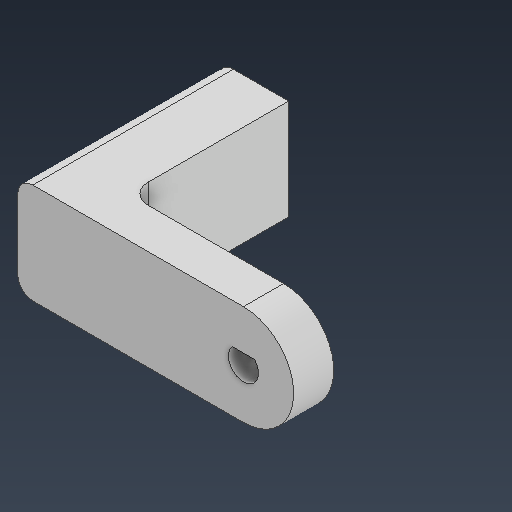
# Autodesk Inventor part: AcoplePPR
Saved by Autodesk Inventor 2027 (Build 310192000, 192)
## iProperties
Created: 2026-08-17
Part Number: AcoplePPR
Material: Generic
Document SubType Name: Modeling
Designer: 06aar
Density: 1 g/cm^3
Appearance: Default
Author: 06aar
Autodesk Inventor part; units mm, degrees
ref_plane "YZ Plane" through (0, 0, 0) normal (1, 0, 0) x (0, 1, 0)
ref_plane "XZ Plane" through (0, 0, 0) normal (0, 1, 0) x (-1, 0, 0)
ref_plane "XY Plane" through (0, 0, 0) normal (0, 0, 1) x (1, 0, 0)
sketch "Sketch1" plane through (0, 0, 0) normal (0, 0, 1) x (1, 0, 0)
  circle A0 centre (0, 0) radius 1.5
  circle A1 centre (0, 0) radius 5
  line L0 (0, 5) -> (-17.5, 5)
  circle A2 centre (-17.5, 0) radius 5
  line L1 (-17.5, -5) -> (0, -5)
  line L2 (-17.5, 0) -> (0, 0)
  line L3 (-17.5, 5) -> (-22.5, 5)
  line L4 (-22.5, 5) -> (-22.5, -5)
  line L5 (-22.5, -5) -> (-17.5, -5)
  line L6 (-1.118, 1) -> (1.118, 1)
  line L7 (0, 1) -> (0, -1.5)
  point P0 (-22.5, 0)
  dimension "d0" = 3
  dimension "d1" = 3.5
  dimension "d3" = 17.5
  dimension "d12" = 2.5
  constraints: 16 end point, 7 point on circle, 6 tangent, 4 horizontal, 3 centre point, 2 coincident, 2 perpendicular, 1 midpoint, 1 parallel, 1 vertical
  measures "d0" diameter of A0
  measures "d1" radial gap between concentric circles of A0 A1
  measures "d3" distance of point (0, 0) L2.start
  measures "d12" distance of L7.start L7.end
extrude "Extrusion1" add sketch "Sketch1" along normal blind 4 contours A1 | A1 L1 A2 L2 | L2 A2 L0 A1 | L6 A0 | A2 | A2 L4 L3 | L5 L4 A2
fillet "Fillet1" radius 1.5 2 edges at (-22.5, 5, 2) (-22.5, -5, 2)
sketch "Sketch3" plane through (0, 0, 0) normal (0, 0, -1) x (-1, 0, 0)
  arc A0 (21, -5) -> (22.5, -3.5) centre (21, -3.5) ccw projected
  line L0 (21, -5) -> (0, -5) projected
  arc A1 (0, 5) -> (0, -5) centre (0, 0) ccw projected
  line L1 (0, 5) -> (21, 5) projected
  arc A2 (22.5, 3.5) -> (21, 5) centre (21, 3.5) ccw projected
  line L2 (22.5, 3.5) -> (22.5, -3.5) projected
  arc A3 (-1.118, 1) -> (1.118, 1) centre (0, 0) ccw projected
  line L3 (0, 5) -> (21, 5) projected
  arc A4 (22.5, 3.5) -> (21, 5) centre (21, 3.5) ccw projected
  line L4 (15.5, 5) -> (15.5, -5)
  line L5 (21, -5) -> (0, -5) projected
  line L6 (1.118, 1) -> (-1.118, 1) projected
  dimension "d8" = 7
  constraints: 2 end point, 2 point on line
  measures "d8" distance between parallel lines of L2 L4
extrude "Extrusion2" add sketch "Sketch3" along normal blind 16 contours L0 L4 L1 A2 L2 A0
fillet "Fillet2" radius 2 1 edges at (-15.5, 0, 0)
body "Solid1"
